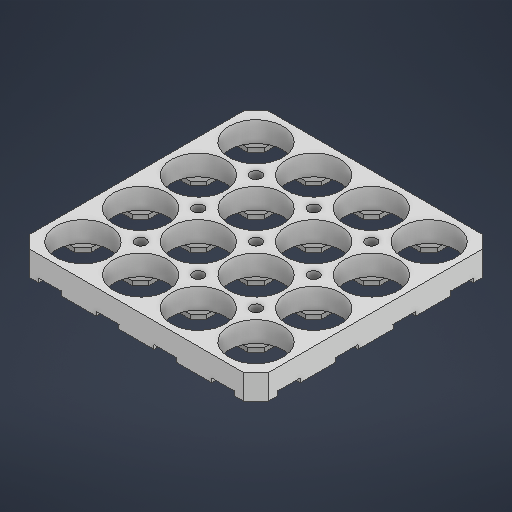
# Autodesk Inventor part: battery_pack_16s
Saved by Autodesk Inventor 2026.1 (Build 301233000, 233)
## iProperties
Created: 2026-03-08
Part Number: battery_pack_16s
Material: Generic
Document SubType Name: Modeling
Designer: aaron
Density: 1 g/cm^3
Appearance: Default
Author: aaron
Autodesk Inventor part; units mm, degrees
ref_plane "YZ Plane" through (0, 0, 0) normal (1, 0, 0) x (0, 1, 0)
ref_plane "XZ Plane" through (0, 0, 0) normal (0, 1, 0) x (-1, 0, 0)
ref_plane "XY Plane" through (0, 0, 0) normal (0, 0, 1) x (1, 0, 0)
sketch "Sketch1" plane through (0, 0, 0) normal (0, 1, 0) x (-1, 0, 0)
  circle A0 centre (10.7499, 10.3753) radius 13.1
  line L0 (10.7499, 10.3753) -> (10.7499, 16.4412)
  line L1 (10.7499, 10.3753) -> (17.5689, 10.3753)
  circle A1 centre (10.7499, 38.3753) radius 13.1
  circle A2 centre (10.7499, 66.3753) radius 13.1
  circle A3 centre (10.7499, 94.3753) radius 13.1
  circle A4 centre (38.7499, 10.3753) radius 13.1
  circle A5 centre (38.7499, 38.3753) radius 13.1
  circle A6 centre (38.7499, 66.3753) radius 13.1
  circle A7 centre (38.7499, 94.3753) radius 13.1
  circle A8 centre (66.7499, 10.3753) radius 13.1
  circle A9 centre (66.7499, 38.3753) radius 13.1
  circle A10 centre (66.7499, 66.3753) radius 13.1
  circle A11 centre (66.7499, 94.3753) radius 13.1
  circle A12 centre (94.7499, 10.3753) radius 13.1
  circle A13 centre (94.7499, 38.3753) radius 13.1
  circle A14 centre (94.7499, 66.3753) radius 13.1
  circle A15 centre (94.7499, 94.3753) radius 13.1
  line L2 (110.7499, 110.3753) -> (-5.2501, 110.3753)
  line L3 (-5.2501, 110.3753) -> (-5.2501, -5.6247)
  line L4 (-5.2501, -5.6247) -> (110.7499, -5.6247)
  line L5 (110.7499, -5.6247) -> (110.7499, 110.3753)
  point P0 (0, 0)
  dimension "d0" = 26.2
  dimension "d3" = 28
  dimension "d6" = 28
  dimension "d9" = 16
  dimension "d10" = 16
  dimension "d11" = 16
  dimension "d12" = 16
  constraints: 16 centre point, 12 end point, 3 horizontal, 2 parallel, 2 vertical, 1 perpendicular, 30 other
  measures "d0" diameter of A0
  measures "d3" distance of L0.start A1.centre
  measures "d6" distance of L0.start A4.centre
  measures "d9" distance from line of L5 A15.centre
  measures "d10" distance from line of L3 A3.centre
  measures "d11" distance from line of L2 A15.centre
  measures "d12" distance from line of L4 A12.centre
extrude "Extrusion1" add sketch "Sketch1" along normal blind 10
sketch "Sketch2" plane through (0, 0, 0) normal (0, -1, 0) x (1, 0, 0)
  line L0 (-110.7499, 110.3753) -> (5.2501, 110.3753) projected
  line L1 (5.2501, 110.3753) -> (5.2501, -5.6247) projected
  line L2 (5.2501, -5.6247) -> (-110.7499, -5.6247) projected
  line L3 (-110.7499, -5.6247) -> (-110.7499, 110.3753) projected
  circle A0 centre (-10.7499, 94.3753) radius 13.1 projected
  circle A1 centre (-10.7499, 10.3753) radius 13.1 projected
  line L4 (7.7501, 116.8753) -> (-1.2499, 116.8753)
  line L5 (-5.2499, 112.8753) -> (-5.2499, 103.8753)
  line L6 (-1.2499, 99.8753) -> (7.7501, 99.8753)
  line L7 (11.7501, 103.8753) -> (11.7501, 112.8753)
  line L8 (-10.7499, 94.3753) -> (15.2741, 94.3753)
  line L9 (-10.7499, 94.3753) -> (-10.7499, 120.6276)
  circle A2 centre (-38.7499, 94.3753) radius 13.1 projected
  circle A3 centre (-38.7499, 66.3753) radius 13.1 projected
  line L10 (-38.7499, 94.3753) -> (-38.7499, 66.3753)
  circle A4 centre (-66.7499, 66.3753) radius 13.1 projected
  line L11 (-38.7499, 66.3753) -> (-66.7499, 66.3753)
  line L12 (-5.2499, 103.8753) -> (-1.2499, 99.8753)
  line L13 (-1.2499, 116.8753) -> (-5.2499, 112.8753)
  line L14 (7.7501, 116.8753) -> (11.7501, 112.8753)
  line L15 (7.7501, 99.8753) -> (11.7501, 103.8753)
  line L16 (7.7501, 88.8753) -> (11.7501, 84.8753)
  line L17 (11.7501, 75.8753) -> (11.7501, 84.8753)
  line L18 (7.7501, 88.8753) -> (-1.2499, 88.8753)
  line L19 (-1.2499, 88.8753) -> (-5.2499, 84.8753)
  line L20 (-5.2499, 84.8753) -> (-5.2499, 75.8753)
  line L21 (-5.2499, 75.8753) -> (-1.2499, 71.8753)
  line L22 (-1.2499, 71.8753) -> (7.7501, 71.8753)
  line L23 (7.7501, 71.8753) -> (11.7501, 75.8753)
  line L24 (7.7501, 60.8753) -> (11.7501, 56.8753)
  line L25 (11.7501, 47.8753) -> (11.7501, 56.8753)
  line L26 (7.7501, 60.8753) -> (-1.2499, 60.8753)
  line L27 (-1.2499, 60.8753) -> (-5.2499, 56.8753)
  line L28 (-5.2499, 56.8753) -> (-5.2499, 47.8753)
  line L29 (-5.2499, 47.8753) -> (-1.2499, 43.8753)
  line L30 (-1.2499, 43.8753) -> (7.7501, 43.8753)
  line L31 (7.7501, 43.8753) -> (11.7501, 47.8753)
  line L32 (7.7501, 32.8753) -> (11.7501, 28.8753)
  line L33 (11.7501, 19.8753) -> (11.7501, 28.8753)
  line L34 (7.7501, 32.8753) -> (-1.2499, 32.8753)
  line L35 (-1.2499, 32.8753) -> (-5.2499, 28.8753)
  line L36 (-5.2499, 28.8753) -> (-5.2499, 19.8753)
  line L37 (-5.2499, 19.8753) -> (-1.2499, 15.8753)
  line L38 (-1.2499, 15.8753) -> (7.7501, 15.8753)
  line L39 (7.7501, 15.8753) -> (11.7501, 19.8753)
  line L40 (7.7501, 4.8753) -> (11.7501, 0.8753)
  line L41 (11.7501, -8.1247) -> (11.7501, 0.8753)
  line L42 (7.7501, 4.8753) -> (-1.2499, 4.8753)
  line L43 (-1.2499, 4.8753) -> (-5.2499, 0.8753)
  line L44 (-5.2499, 0.8753) -> (-5.2499, -8.1247)
  line L45 (-5.2499, -8.1247) -> (-1.2499, -12.1247)
  line L46 (-1.2499, -12.1247) -> (7.7501, -12.1247)
  line L47 (7.7501, -12.1247) -> (11.7501, -8.1247)
  line L48 (-20.2499, 116.8753) -> (-16.2499, 112.8753)
  line L49 (-16.2499, 103.8753) -> (-16.2499, 112.8753)
  line L50 (-20.2499, 116.8753) -> (-29.2499, 116.8753)
  line L51 (-29.2499, 116.8753) -> (-33.2499, 112.8753)
  line L52 (-33.2499, 112.8753) -> (-33.2499, 103.8753)
  line L53 (-33.2499, 103.8753) -> (-29.2499, 99.8753)
  line L54 (-29.2499, 99.8753) -> (-20.2499, 99.8753)
  line L55 (-20.2499, 99.8753) -> (-16.2499, 103.8753)
  line L56 (-20.2499, 88.8753) -> (-16.2499, 84.8753)
  line L57 (-16.2499, 75.8753) -> (-16.2499, 84.8753)
  line L58 (-20.2499, 88.8753) -> (-29.2499, 88.8753)
  line L59 (-29.2499, 88.8753) -> (-33.2499, 84.8753)
  line L60 (-33.2499, 84.8753) -> (-33.2499, 75.8753)
  line L61 (-33.2499, 75.8753) -> (-29.2499, 71.8753)
  line L62 (-29.2499, 71.8753) -> (-20.2499, 71.8753)
  line L63 (-20.2499, 71.8753) -> (-16.2499, 75.8753)
  line L64 (-20.2499, 60.8753) -> (-16.2499, 56.8753)
  line L65 (-16.2499, 47.8753) -> (-16.2499, 56.8753)
  line L66 (-20.2499, 60.8753) -> (-29.2499, 60.8753)
  line L67 (-29.2499, 60.8753) -> (-33.2499, 56.8753)
  line L68 (-33.2499, 56.8753) -> (-33.2499, 47.8753)
  line L69 (-33.2499, 47.8753) -> (-29.2499, 43.8753)
  line L70 (-29.2499, 43.8753) -> (-20.2499, 43.8753)
  line L71 (-20.2499, 43.8753) -> (-16.2499, 47.8753)
  line L72 (-20.2499, 32.8753) -> (-16.2499, 28.8753)
  line L73 (-16.2499, 19.8753) -> (-16.2499, 28.8753)
  line L74 (-20.2499, 32.8753) -> (-29.2499, 32.8753)
  line L75 (-29.2499, 32.8753) -> (-33.2499, 28.8753)
  line L76 (-33.2499, 28.8753) -> (-33.2499, 19.8753)
  line L77 (-33.2499, 19.8753) -> (-29.2499, 15.8753)
  line L78 (-29.2499, 15.8753) -> (-20.2499, 15.8753)
  line L79 (-20.2499, 15.8753) -> (-16.2499, 19.8753)
  line L80 (-20.2499, 4.8753) -> (-16.2499, 0.8753)
  line L81 (-16.2499, -8.1247) -> (-16.2499, 0.8753)
  line L82 (-20.2499, 4.8753) -> (-29.2499, 4.8753)
  line L83 (-29.2499, 4.8753) -> (-33.2499, 0.8753)
  line L84 (-33.2499, 0.8753) -> (-33.2499, -8.1247)
  line L85 (-33.2499, -8.1247) -> (-29.2499, -12.1247)
  line L86 (-29.2499, -12.1247) -> (-20.2499, -12.1247)
  line L87 (-20.2499, -12.1247) -> (-16.2499, -8.1247)
  line L88 (-48.2499, 116.8753) -> (-44.2499, 112.8753)
  line L89 (-44.2499, 103.8753) -> (-44.2499, 112.8753)
  line L90 (-48.2499, 116.8753) -> (-57.2499, 116.8753)
  line L91 (-57.2499, 116.8753) -> (-61.2499, 112.8753)
  line L92 (-61.2499, 112.8753) -> (-61.2499, 103.8753)
  line L93 (-61.2499, 103.8753) -> (-57.2499, 99.8753)
  line L94 (-57.2499, 99.8753) -> (-48.2499, 99.8753)
  line L95 (-48.2499, 99.8753) -> (-44.2499, 103.8753)
  line L96 (-48.2499, 88.8753) -> (-44.2499, 84.8753)
  line L97 (-44.2499, 75.8753) -> (-44.2499, 84.8753)
  line L98 (-48.2499, 88.8753) -> (-57.2499, 88.8753)
  line L99 (-57.2499, 88.8753) -> (-61.2499, 84.8753)
  line L100 (-61.2499, 84.8753) -> (-61.2499, 75.8753)
  line L101 (-61.2499, 75.8753) -> (-57.2499, 71.8753)
  line L102 (-57.2499, 71.8753) -> (-48.2499, 71.8753)
  line L103 (-48.2499, 71.8753) -> (-44.2499, 75.8753)
  line L104 (-48.2499, 60.8753) -> (-44.2499, 56.8753)
  line L105 (-44.2499, 47.8753) -> (-44.2499, 56.8753)
  line L106 (-48.2499, 60.8753) -> (-57.2499, 60.8753)
  line L107 (-57.2499, 60.8753) -> (-61.2499, 56.8753)
  line L108 (-61.2499, 56.8753) -> (-61.2499, 47.8753)
  line L109 (-61.2499, 47.8753) -> (-57.2499, 43.8753)
  line L110 (-57.2499, 43.8753) -> (-48.2499, 43.8753)
  line L111 (-48.2499, 43.8753) -> (-44.2499, 47.8753)
  line L112 (-48.2499, 32.8753) -> (-44.2499, 28.8753)
  line L113 (-44.2499, 19.8753) -> (-44.2499, 28.8753)
  line L114 (-48.2499, 32.8753) -> (-57.2499, 32.8753)
  line L115 (-57.2499, 32.8753) -> (-61.2499, 28.8753)
  line L116 (-61.2499, 28.8753) -> (-61.2499, 19.8753)
  line L117 (-61.2499, 19.8753) -> (-57.2499, 15.8753)
  line L118 (-57.2499, 15.8753) -> (-48.2499, 15.8753)
  line L119 (-48.2499, 15.8753) -> (-44.2499, 19.8753)
  line L120 (-48.2499, 4.8753) -> (-44.2499, 0.8753)
  line L121 (-44.2499, -8.1247) -> (-44.2499, 0.8753)
  line L122 (-48.2499, 4.8753) -> (-57.2499, 4.8753)
  line L123 (-57.2499, 4.8753) -> (-61.2499, 0.8753)
  line L124 (-61.2499, 0.8753) -> (-61.2499, -8.1247)
  line L125 (-61.2499, -8.1247) -> (-57.2499, -12.1247)
  line L126 (-57.2499, -12.1247) -> (-48.2499, -12.1247)
  line L127 (-48.2499, -12.1247) -> (-44.2499, -8.1247)
  line L128 (-76.2499, 116.8753) -> (-72.2499, 112.8753)
  line L129 (-72.2499, 103.8753) -> (-72.2499, 112.8753)
  line L130 (-76.2499, 116.8753) -> (-85.2499, 116.8753)
  line L131 (-85.2499, 116.8753) -> (-89.2499, 112.8753)
  line L132 (-89.2499, 112.8753) -> (-89.2499, 103.8753)
  line L133 (-89.2499, 103.8753) -> (-85.2499, 99.8753)
  line L134 (-85.2499, 99.8753) -> (-76.2499, 99.8753)
  line L135 (-76.2499, 99.8753) -> (-72.2499, 103.8753)
  line L136 (-76.2499, 88.8753) -> (-72.2499, 84.8753)
  line L137 (-72.2499, 75.8753) -> (-72.2499, 84.8753)
  line L138 (-76.2499, 88.8753) -> (-85.2499, 88.8753)
  line L139 (-85.2499, 88.8753) -> (-89.2499, 84.8753)
  line L140 (-89.2499, 84.8753) -> (-89.2499, 75.8753)
  line L141 (-89.2499, 75.8753) -> (-85.2499, 71.8753)
  line L142 (-85.2499, 71.8753) -> (-76.2499, 71.8753)
  line L143 (-76.2499, 71.8753) -> (-72.2499, 75.8753)
  line L144 (-76.2499, 60.8753) -> (-72.2499, 56.8753)
  line L145 (-72.2499, 47.8753) -> (-72.2499, 56.8753)
  line L146 (-76.2499, 60.8753) -> (-85.2499, 60.8753)
  line L147 (-85.2499, 60.8753) -> (-89.2499, 56.8753)
  line L148 (-89.2499, 56.8753) -> (-89.2499, 47.8753)
  line L149 (-89.2499, 47.8753) -> (-85.2499, 43.8753)
  line L150 (-85.2499, 43.8753) -> (-76.2499, 43.8753)
  line L151 (-76.2499, 43.8753) -> (-72.2499, 47.8753)
  line L152 (-76.2499, 32.8753) -> (-72.2499, 28.8753)
  line L153 (-72.2499, 19.8753) -> (-72.2499, 28.8753)
  line L154 (-76.2499, 32.8753) -> (-85.2499, 32.8753)
  line L155 (-85.2499, 32.8753) -> (-89.2499, 28.8753)
  line L156 (-89.2499, 28.8753) -> (-89.2499, 19.8753)
  line L157 (-89.2499, 19.8753) -> (-85.2499, 15.8753)
  line L158 (-85.2499, 15.8753) -> (-76.2499, 15.8753)
  line L159 (-76.2499, 15.8753) -> (-72.2499, 19.8753)
  line L160 (-76.2499, 4.8753) -> (-72.2499, 0.8753)
  line L161 (-72.2499, -8.1247) -> (-72.2499, 0.8753)
  line L162 (-76.2499, 4.8753) -> (-85.2499, 4.8753)
  line L163 (-85.2499, 4.8753) -> (-89.2499, 0.8753)
  line L164 (-89.2499, 0.8753) -> (-89.2499, -8.1247)
  line L165 (-89.2499, -8.1247) -> (-85.2499, -12.1247)
  line L166 (-85.2499, -12.1247) -> (-76.2499, -12.1247)
  line L167 (-76.2499, -12.1247) -> (-72.2499, -8.1247)
  line L168 (-104.2499, 116.8753) -> (-100.2499, 112.8753)
  line L169 (-100.2499, 103.8753) -> (-100.2499, 112.8753)
  line L170 (-104.2499, 116.8753) -> (-113.2499, 116.8753)
  line L171 (-113.2499, 116.8753) -> (-117.2499, 112.8753)
  line L172 (-117.2499, 112.8753) -> (-117.2499, 103.8753)
  line L173 (-117.2499, 103.8753) -> (-113.2499, 99.8753)
  line L174 (-113.2499, 99.8753) -> (-104.2499, 99.8753)
  line L175 (-104.2499, 99.8753) -> (-100.2499, 103.8753)
  line L176 (-104.2499, 88.8753) -> (-100.2499, 84.8753)
  line L177 (-100.2499, 75.8753) -> (-100.2499, 84.8753)
  line L178 (-104.2499, 88.8753) -> (-113.2499, 88.8753)
  line L179 (-113.2499, 88.8753) -> (-117.2499, 84.8753)
  line L180 (-117.2499, 84.8753) -> (-117.2499, 75.8753)
  line L181 (-117.2499, 75.8753) -> (-113.2499, 71.8753)
  line L182 (-113.2499, 71.8753) -> (-104.2499, 71.8753)
  line L183 (-104.2499, 71.8753) -> (-100.2499, 75.8753)
  line L184 (-104.2499, 60.8753) -> (-100.2499, 56.8753)
  line L185 (-100.2499, 47.8753) -> (-100.2499, 56.8753)
  line L186 (-104.2499, 60.8753) -> (-113.2499, 60.8753)
  line L187 (-113.2499, 60.8753) -> (-117.2499, 56.8753)
  line L188 (-117.2499, 56.8753) -> (-117.2499, 47.8753)
  line L189 (-117.2499, 47.8753) -> (-113.2499, 43.8753)
  line L190 (-113.2499, 43.8753) -> (-104.2499, 43.8753)
  line L191 (-104.2499, 43.8753) -> (-100.2499, 47.8753)
  line L192 (-104.2499, 32.8753) -> (-100.2499, 28.8753)
  line L193 (-100.2499, 19.8753) -> (-100.2499, 28.8753)
  line L194 (-104.2499, 32.8753) -> (-113.2499, 32.8753)
  line L195 (-113.2499, 32.8753) -> (-117.2499, 28.8753)
  line L196 (-117.2499, 28.8753) -> (-117.2499, 19.8753)
  line L197 (-117.2499, 19.8753) -> (-113.2499, 15.8753)
  line L198 (-113.2499, 15.8753) -> (-104.2499, 15.8753)
  line L199 (-104.2499, 15.8753) -> (-100.2499, 19.8753)
  line L200 (-104.2499, 4.8753) -> (-100.2499, 0.8753)
  line L201 (-100.2499, -8.1247) -> (-100.2499, 0.8753)
  line L202 (-104.2499, 4.8753) -> (-113.2499, 4.8753)
  line L203 (-113.2499, 4.8753) -> (-117.2499, 0.8753)
  line L204 (-117.2499, 0.8753) -> (-117.2499, -8.1247)
  line L205 (-117.2499, -8.1247) -> (-113.2499, -12.1247)
  line L206 (-113.2499, -12.1247) -> (-104.2499, -12.1247)
  line L207 (-104.2499, -12.1247) -> (-100.2499, -8.1247)
  circle A5 centre (-94.7499, 10.3753) radius 13.1 projected
  circle A6 centre (-94.7499, 38.3753) radius 13.1 projected
  circle A7 centre (-94.7499, 66.3753) radius 13.1 projected
  circle A8 centre (-94.7499, 94.3753) radius 13.1 projected
  circle A9 centre (-66.7499, 94.3753) radius 13.1 projected
  circle A10 centre (-66.7499, 38.3753) radius 13.1 projected
  circle A11 centre (-38.7499, 38.3753) radius 13.1 projected
  circle A12 centre (-66.7499, 10.3753) radius 13.1 projected
  circle A13 centre (-38.7499, 10.3753) radius 13.1 projected
  circle A14 centre (-10.7499, 38.3753) radius 13.1 projected
  circle A15 centre (-10.7499, 66.3753) radius 13.1 projected
  point P0 (11.7501, 116.8753)
  point P1 (-5.2499, 99.8753)
  point P2 (-5.2499, 116.8753)
  point P3 (11.7501, 99.8753)
  point P4 (-72.2499, -5.6247)
  point P5 (-78.6394, 4.8753)
  point P6 (-78.6394, 15.8753)
  point P7 (-72.2499, 22.2648)
  point P8 (-61.2499, 22.2648)
  point P9 (-54.8604, 15.8753)
  point P10 (-54.8604, 4.8753)
  point P11 (-61.2499, -5.6247)
  point P12 (1.1396, 99.8753)
  point P13 (1.1396, 88.8753)
  point P14 (-5.2499, 82.4858)
  point P15 (-16.2499, 82.4858)
  point P16 (-22.6394, 88.8753)
  point P17 (-22.6394, 99.8753)
  point P18 (-16.2499, 106.2648)
  point P19 (-5.2499, 106.2648)
  point P20 (1.1396, 4.8753)
  point P21 (-5.2499, -1.5142)
  point P22 (-16.2499, -1.5142)
  point P23 (-22.6394, 4.8753)
  point P24 (-22.6394, 15.8753)
  point P25 (-16.2499, 22.2648)
  point P26 (-5.2499, 22.2648)
  point P27 (1.1396, 15.8753)
  point P28 (-26.8604, 99.8753)
  point P29 (-26.8604, 88.8753)
  point P30 (-33.2499, 82.4858)
  point P31 (-44.2499, 82.4858)
  point P32 (-50.6394, 88.8753)
  point P33 (-50.6394, 99.8753)
  point P34 (-44.2499, 106.2648)
  point P35 (-33.2499, 106.2648)
  point P36 (-33.2499, 78.2648)
  point P37 (-26.8604, 71.8753)
  point P38 (-26.8604, 60.8753)
  point P39 (-33.2499, 54.4858)
  point P40 (-44.2499, 54.4858)
  point P41 (-50.6394, 60.8753)
  point P42 (-50.6394, 71.8753)
  point P43 (-44.2499, 78.2648)
  point P44 (-54.8604, 60.8753)
  point P45 (-61.2499, 54.4858)
  point P46 (-72.2499, 54.4858)
  point P47 (-78.6394, 60.8753)
  point P48 (-78.6394, 71.8753)
  point P49 (-72.2499, 78.2648)
  point P50 (-61.2499, 78.2648)
  point P51 (-54.8604, 71.8753)
  point P52 (-100.2499, -1.5142)
  point P53 (-106.6394, 4.8753)
  point P54 (-106.6394, 15.8753)
  point P55 (-100.2499, 22.2648)
  point P56 (-89.2499, 22.2648)
  point P57 (-82.8604, 15.8753)
  point P58 (-82.8604, 4.8753)
  point P59 (-89.2499, -1.5142)
  point P60 (-100.2499, 26.4858)
  point P61 (-106.6394, 32.8753)
  point P62 (-106.6394, 43.8753)
  point P63 (-100.2499, 50.2648)
  point P64 (-89.2499, 50.2648)
  point P65 (-82.8604, 43.8753)
  point P66 (-82.8604, 32.8753)
  point P67 (-89.2499, 26.4858)
  point P68 (-100.2499, 106.2648)
  point P69 (-89.2499, 106.2648)
  point P70 (-82.8604, 99.8753)
  point P71 (-82.8604, 88.8753)
  point P72 (-89.2499, 82.4858)
  point P73 (-100.2499, 82.4858)
  point P74 (-106.6394, 88.8753)
  point P75 (-106.6394, 99.8753)
  point P76 (-54.8604, 99.8753)
  point P77 (-54.8604, 88.8753)
  point P78 (-61.2499, 82.4858)
  point P79 (-72.2499, 82.4858)
  point P80 (-78.6394, 88.8753)
  point P81 (-78.6394, 99.8753)
  point P82 (-72.2499, 106.2648)
  point P83 (-61.2499, 106.2648)
  point P84 (-44.2499, 22.2648)
  point P85 (-33.2499, 22.2648)
  point P86 (-26.8604, 15.8753)
  point P87 (-26.8604, 4.8753)
  point P88 (-33.2499, -1.5142)
  point P89 (-44.2499, -1.5142)
  point P90 (-50.6394, 4.8753)
  point P91 (-50.6394, 15.8753)
  point P92 (1.1396, 71.8753)
  point P93 (1.1396, 60.8753)
  point P94 (-5.2499, 54.4858)
  point P95 (-16.2499, 54.4858)
  point P96 (-22.6394, 60.8753)
  point P97 (-22.6394, 71.8753)
  point P98 (-16.2499, 78.2648)
  point P99 (-5.2499, 78.2648)
  point P100 (1.1396, 32.8753)
  point P101 (-5.2499, 26.4858)
  point P102 (-16.2499, 26.4858)
  point P103 (-22.6394, 32.8753)
  point P104 (-22.6394, 43.8753)
  point P105 (-16.2499, 50.2648)
  point P106 (-5.2499, 50.2648)
  point P107 (1.1396, 43.8753)
  point P108 (-50.6394, 43.8753)
  point P109 (-44.2499, 50.2648)
  point P110 (-33.2499, 50.2648)
  point P111 (-26.8604, 43.8753)
  point P112 (-26.8604, 32.8753)
  point P113 (-33.2499, 26.4858)
  point P114 (-44.2499, 26.4858)
  point P115 (-50.6394, 32.8753)
  point P116 (-78.6394, 43.8753)
  point P117 (-72.2499, 50.2648)
  point P118 (-61.2499, 50.2648)
  point P119 (-54.8604, 43.8753)
  point P120 (-54.8604, 32.8753)
  point P121 (-61.2499, 26.4858)
  point P122 (-72.2499, 26.4858)
  point P123 (-78.6394, 32.8753)
  point P124 (-100.2499, 54.4858)
  point P125 (-106.6394, 60.8753)
  point P126 (-106.6394, 71.8753)
  point P127 (-100.2499, 78.2648)
  point P128 (-89.2499, 78.2648)
  point P129 (-82.8604, 71.8753)
  point P130 (-82.8604, 60.8753)
  point P131 (-89.2499, 54.4858)
  point P132 (-61.2499, -1.5142)
  point P133 (-72.2499, -1.5142)
  point P134 (5.2501, 99.8753)
  point P135 (-5.2499, 110.3753)
  point P136 (5.2501, 71.8753)
  point P137 (5.2501, 88.8753)
  point P138 (-110.7499, 4.8753)
  point P139 (-100.2499, -5.6247)
  point P140 (-110.7499, 32.8753)
  point P141 (-110.7499, 15.8753)
  point P142 (-110.7499, 60.8753)
  point P143 (-110.7499, 43.8753)
  point P144 (-100.2499, 110.3753)
  point P145 (-110.7499, 99.8753)
  point P146 (-110.7499, 88.8753)
  point P147 (-110.7499, 71.8753)
  point P148 (-89.2499, -5.6247)
  point P149 (-72.2499, 110.3753)
  point P150 (-89.2499, 110.3753)
  point P151 (-44.2499, -5.6247)
  point P152 (-44.2499, 110.3753)
  point P153 (-61.2499, 110.3753)
  point P154 (-5.2499, -5.6247)
  point P155 (5.2501, 4.8753)
  point P156 (-33.2499, -5.6247)
  point P157 (-16.2499, -5.6247)
  point P158 (5.2501, 15.8753)
  point P159 (5.2501, 32.8753)
  point P160 (5.2501, 43.8753)
  point P161 (5.2501, 60.8753)
  point P162 (-16.2499, 110.3753)
  point P163 (-33.2499, 110.3753)
  dimension "d19" = 17
  dimension "d20" = 17
  dimension "d21" = 5.5
  dimension "d22" = 28
  dimension "d23" = 5.5
  dimension "d24" = 4
  dimension "d25" = 4
  dimension "d26" = 4
  dimension "d27" = 4
  dimension "d28" = 4
  dimension "d29" = 4
  dimension "d30" = 4
  dimension "d31" = 4
  dimension "d34" = 28
  dimension "d37" = 28
  constraints: 408 end point, 8 point on line, 3 horizontal, 3 vertical, 2 parallel, 2 perpendicular, 384 other
  measures "d19" distance of point (11.75, 116.875) point (-5.25, 116.875)
  measures "d20" distance of point (11.75, 99.875) point (11.75, 116.875)
  measures "d21" distance between parallel lines of L8 L6
  measures "d22" distance of L10.start L10.end
  measures "d23" distance between parallel lines of L9 L5
  measures "d24" distance of L5.end point (-5.25, 99.875)
  measures "d25" distance of L6.start point (-5.25, 99.875)
  measures "d26" distance of L4.end point (-5.25, 116.875)
  measures "d27" distance of L5.start point (-5.25, 116.875)
  measures "d28" distance of L4.start point (11.75, 116.875)
  measures "d29" distance of L7.end point (11.75, 116.875)
  measures "d30" distance of L6.end point (11.75, 99.875)
  measures "d31" distance of L7.start point (11.75, 99.875)
  measures "d34" distance of L4.start L16.start
  measures "d37" distance of L4.start L48.start
extrude "Extrusion2" add sketch "Sketch2" along normal blind 2 contours L0 L169 A8 L174 L3 | L0 L129 A9 L134 A8 L132 | L169 L175 L174 A8 | L178 A8 L177 A7 L182 L3 | A8 L134 L133 L132 | L178 L176 L177 A8 | L0 L89 A2 L94 A9 L92 | L129 L135 L134 A9 | L186 A7 L185 A6 L190 L3 | A7 L177 L183 L182 | A9 L94 L93 L92 | L186 L184 L185 A7 | A8 L138 A9 L137 A4 L142 A7 L140 | L140 L139 L138 A8 | L0 L49 A0 L54 A2 L52 | L89 L95 L94 A2 | L138 L136 L137 A9 | L194 A6 L193 A5 L198 L3 | A6 L185 L191 L190 | A7 L142 L141 L140 | A2 L54 L53 L52 | L194 L192 L193 A6 | A7 L146 A4 L145 A10 L150 A6 L148 | L148 L147 L146 A7 | L49 L55 L54 A0 | L98 L96 L97 A2 | A2 L97 A3 L102 A4 L100 A9 L98 | A9 L100 L99 L98 | L137 L143 L142 A4 | L202 A5 L201 L2 L3 | A5 L193 L199 L198 | A6 L150 L149 L148 | L0 L1 L6 A0 L5 | A4 L102 L101 L100 | L202 L200 L201 A5 | A6 L154 A10 L153 A12 L158 A5 L156 | L156 L155 L154 A6 | L146 L144 L145 A4 | A0 L6 L12 L5 | L58 L56 L57 A0 | A0 L57 A15 L62 A3 L60 A2 L58 | A2 L60 L59 L58 | L97 L103 L102 A3 | A5 L158 L157 L156 | A10 L145 L151 L150 | L164 A5 L162 A12 L161 L2 | L164 L163 L162 A5 | L154 L152 L153 A10 | L108 L107 L106 A4 | A4 L106 A3 L105 A11 L110 A10 L108 | L18 L1 L22 A15 L20 A0 | A0 L20 L19 L18 | L57 L63 L62 A15 | A3 L62 L61 L60 | A12 L153 L159 L158 | A10 L110 L109 L108 | A15 L22 L21 L20 | L106 L104 L105 A3 | L124 A12 L122 A13 L121 L2 | A12 L162 L160 L161 | A10 L114 A11 L113 A13 L118 A12 L116 | L116 L115 L114 A10 | A15 L65 A14 L70 A11 L68 A3 L66 | L66 L64 L65 A15 | L124 L123 L122 A12 | A12 L118 L117 L116 | A11 L105 L111 L110 | L1 L30 A14 L28 A15 L26 | A3 L68 L67 L66 | L84 A13 L82 A1 L81 L2 | A13 L122 L120 L121 | L114 L112 L113 A11 | A15 L28 L27 L26 | L65 L71 L70 A14 | A11 L70 L69 L68 | L84 L83 L82 A13 | A13 L113 L119 L118 | L1 L38 A1 L36 A14 L34 | L30 L29 L28 A14 | L44 A1 L42 L1 L2 | A1 L82 L80 L81 | A11 L74 A14 L73 A1 L78 A13 L76 | L76 L75 L74 A11 | A14 L36 L35 L34 | L74 L72 L73 A14 | L44 L43 L42 A1 | A13 L78 L77 L76 | L38 L37 L36 A1 | A1 L73 L79 L78
sketch "Sketch3" plane through (0, -2, 0) normal (0, -1, 0) x (1, 0, 0)
  arc A0 (-33.2499, 78.2648) -> (-44.2499, 78.2648) centre (-38.7499, 66.3753) ccw projected
  circle A1 centre (-38.7499, 38.3753) radius 13.1 projected
  line L0 (-38.7499, 66.3753) -> (-38.7499, 38.3753)
  circle A2 centre (-66.7499, 38.3753) radius 13.1 projected
  line L1 (-38.7499, 38.3753) -> (-66.7499, 38.3753)
  circle A3 centre (-24.7499, 80.3753) radius 2.65
  line L2 (-16.2499, 75.8753) -> (-16.2499, 84.8753) projected
  line L3 (-33.2499, 84.8753) -> (-33.2499, 75.8753) projected
  line L4 (-20.2499, 88.8753) -> (-29.2499, 88.8753) projected
  circle A4 centre (-24.7499, 52.3753) radius 2.65
  circle A5 centre (-24.7499, 24.3753) radius 2.65
  circle A6 centre (-52.7499, 80.3753) radius 2.65
  circle A7 centre (-52.7499, 52.3753) radius 2.65
  circle A8 centre (-52.7499, 24.3753) radius 2.65
  circle A9 centre (-80.7499, 80.3753) radius 2.65
  circle A10 centre (-80.7499, 52.3753) radius 2.65
  circle A11 centre (-80.7499, 24.3753) radius 2.65
  point P0 (0, 0)
  point P1 (-33.2499, 80.3753)
  dimension "d42" = 17
  dimension "d43" = 8.5
  dimension "d44" = 8.5
  dimension "d45" = 5.3
  dimension "d48" = 28
  dimension "d51" = 28
  constraints: 9 centre point, 4 end point, 2 vertical, 1 horizontal, 1 midpoint, 1 perpendicular, 16 other
  measures "d42" distance between parallel lines of L2 L3
  measures "d43" distance of point (-33.25, 80.375) A3.centre
  measures "d44" distance from line of L4 A3.centre
  measures "d45" diameter of A3
  measures "d48" distance of A3.centre A4.centre
  measures "d51" distance of A3.centre A6.centre
extrude "Extrusion3" cut sketch "Sketch3" against normal through all contours A3 | A4 | A5 | A6 | A7 | A8 | A9 | A10 | A11
chamfer "Chamfer1" distance 6 angle 45 4 edges at (5.2501, 4, -5.6247) (5.2501, 4, 110.3753) (-110.7499, 4, 110.3753) (-110.7499, 4, -5.6247)
equation "\"d10\" = d9"
equation "\"d11\" = d9"
equation "\"d12\" = d9"
equation "\"d20\" = d19"
equation "\"d21\" = -0.5 * d20 + 0.5 * d22"
equation "\"d23\" = d21"
equation "\"d25\" = d24"
equation "\"d26\" = d24"
equation "\"d27\" = d26"
equation "\"d28\" = d24"
equation "\"d29\" = d28"
equation "\"d30\" = d24"
equation "\"d31\" = d30"
body "Solid1"
